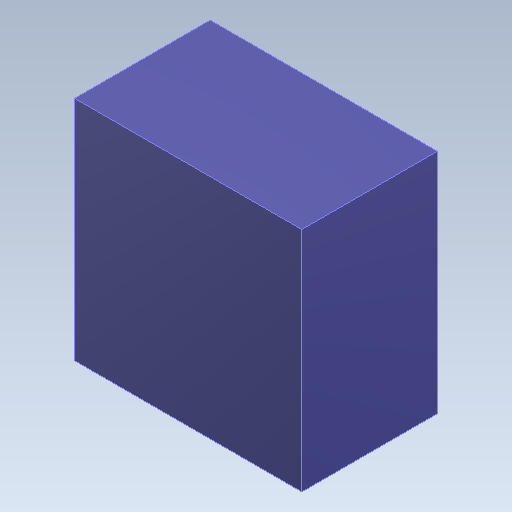
# Autodesk Inventor part: TP_KEYSTONE500X
Saved by Autodesk Inventor 2021 (Build 250183000, 183)
## iProperties
Created: 2020-11-03
Part Number: TP_KEYSTONE500X
Material: Generic
Document SubType Name: Modeling
Designer: faiya
Density: 1 g/cm^3
Appearance: P1_1MM, TP_KEYSTONE500X
Author: faiya
Autodesk Inventor part; units mm, degrees
ref_plane "YZ Plane" through (0, 0, 0) normal (1, 0, 0) x (0, 1, 0)
ref_plane "XZ Plane" through (0, 0, 0) normal (0, 1, 0) x (-1, 0, 0)
ref_plane "XY Plane" through (0, 0, 0) normal (0, 0, 1) x (1, 0, 0)
sketch "P1_1MM, TP_KEYSTONE500X_1" plane through (0, 0, 0) normal (0, 0, 1) x (1, 0, 0)
  line L0 (-0.8382, 0.8382) -> (0.8382, 0.8382)
  line L1 (0.8382, 0.8382) -> (0.8382, -0.8382)
  line L2 (0.8382, -0.8382) -> (-0.8382, -0.8382)
  line L3 (-0.8382, -0.8382) -> (-0.8382, 0.8382)
  constraints: 8 end point
extrude "Extrusion1" add sketch "P1_1MM, TP_KEYSTONE500X_1" along normal blind 1
body "Solid1"
